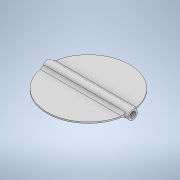
# Autodesk Inventor part: Butterfly valve
Saved by Autodesk Inventor 2020 (Build 240168000, 168)
## iProperties
Created: 2020-04-08
Part Number: Butterfly valve
Material: Generic
Document SubType Name: Modeling
Designer: angusaitken
Density: 1 g/cm^3
Appearance: Default
Author: angusaitken
Autodesk Inventor part; units mm, degrees
ref_plane "YZ Plane" through (0, 0, 0) normal (1, 0, 0) x (0, 1, 0)
ref_plane "XZ Plane" through (0, 0, 0) normal (0, 1, 0) x (-1, 0, 0)
sketch "Sketch1" plane through (0, 0, 0) normal (0, 1, 0) x (-1, 0, 0)
  circle A0 centre (0, 0) radius 38
  dimension "d0" = 76
  constraints: 1 centre point, 1 coincident
  measures "d0" diameter of A0
extrude "Extrusion1" add sketch "Sketch1" along normal blind 1.2
sketch "Sketch2" plane through (0, 0, 0) normal (1, 0, 0) x (0, 1, 0)
  line L0 (1.2, -38) -> (1.2, 38) projected
  line L1 (0, -38) -> (0, 38) projected
  line L2 (0, 38) -> (1.2, 38) projected
  line L3 (0.6, 38) -> (0.6, -38)
  line L4 (0, -38) -> (1.2, -38) projected
  circle A0 centre (0.6, 0) radius 2.825
  circle A1 centre (0.6, 0) radius 4.325
  point P0 (0, 0)
  dimension "d3" = 5.65
  dimension "d4" = 1.5
  constraints: 3 midpoint, 2 centre point, 2 end point
  measures "d3" diameter of A0
  measures "d4" radial gap between concentric circles of A0 A1
extrude "Extrusion2" add sketch "Sketch2" along normal blind 41 contours A1 L3 A0 L0 | L0 A0 A1 | A1 L1 A0 L3 | A0 L3 A1 L0 | A1 L1 A0 | A0 L1 A1 L3
sketch "Sketch3" plane through (0, 0, 0) normal (-1, 0, 0) x (0, 0, 1)
  arc A0 (4.2832, 1.2) -> (-4.2832, 1.2) centre (0, 0.6) ccw projected
  circle A1 centre (0, 0.6) radius 4.325
  point P0 (0, 0)
  point P1 (-4.2832, 1.2)
  constraints: 1 centre point, 1 coincident
extrude "Extrusion3" add sketch "Sketch3" along normal up to surface round surface about axis through (0, 0, 0) along (0, 1, 0) radius 38 far side no
move faces "Move1" translate (33.338, 0, 0) faces at (0, 1.7332, 0.5909) (0, -1.0899, -0.1361)
delete faces "Delete Face1" heal yes whole lump no faces at (37.9988, 0.2662, 0.307) (34.8883, 1.2, -0.307) (34.8883, 0, -0.307)
fillet "Fillet1" radius 4 8 edges at (18.8789, 1.2, -4.2832) (-18.8789, 1.2, -4.2832) (18.8789, 1.2, 4.2832) (-18.8789, 1.2, 4.2832) (18.8789, 0, -4.2832) (-18.8789, 0, -4.2832) (18.8789, 0, 4.2832) (-18.8789, 0, 4.2832)
ref_plane "Work Plane1" through (-38.375, 0.6, 0) normal (1, 0, 0) x (0, 0, -1)
sketch "Sketch4" plane through (-38.375, 0.6, 0) normal (1, 0, 0) x (0, 0, -1)
  line L0 (-6.9387, -0.6) -> (-6.9387, -0.6) projected
  line L1 (-6.9387, 0.6) -> (-6.9387, 0.6) projected
  line L2 (6.9387, 0.6) -> (6.9387, 0.6) projected
  line L3 (6.9387, -0.6) -> (6.9387, -0.6) projected
  point P0 (0, -0.6)
  point P1 (0, 0)
  point P2 (0, 0)
  constraints: 2 horizontal alignment, 2 vertical alignment, 1 coincident, 12 other
hole "Hole1" at (-38.375, 0.6, 0) direction (1, 0, 0) diameter 3.8 depth 25.4 tip angle 118
body "Solid1"
